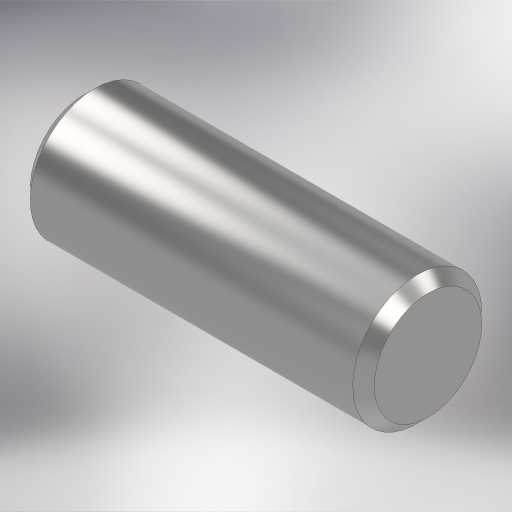
# Autodesk Inventor part: Pin
Saved by Autodesk Inventor 2023 (Build 270158000, 158)
## iProperties
Created: 2023-04-03
Part Number: Pin
Material: Stainless Steel
Document SubType Name: Modeling
Designer: aaron
Density: 8 g/cm^3
Appearance: Semi-Polished
Author: aaron
Autodesk Inventor part; units mm, degrees
ref_plane "YZ Plane" through (0, 0, 0) normal (1, 0, 0) x (0, 1, 0)
ref_plane "XZ Plane" through (0, 0, 0) normal (0, 1, 0) x (-1, 0, 0)
ref_plane "XY Plane" through (0, 0, 0) normal (0, 0, 1) x (1, 0, 0)
sketch "Sketch1" plane through (0, 0, 0) normal (1, 0, 0) x (0, 1, 0)
  circle A0 centre (0, 0) radius 2.3812
  dimension "d0" = 4.7625
  constraints: 1 centre point, 1 coincident
  measures "d0" diameter of A0
extrude "Extrusion1" add sketch "Sketch1" along normal blind 12.7
chamfer "Chamfer1" distance 0.3969 angle 45 2 edges at (12.7, -2.3812, 0) (0, -2.3812, 0)
body "Solid1"
